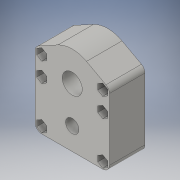
# Autodesk Inventor part: Transmission box
Saved by Autodesk Inventor 2016 SP2 (Build 200236200, 236)
## iProperties
Created: 2018-01-18
Part Number: Transmission box
Material: Generic
Document SubType Name: Modeling
Designer: CAD
Density: 1 g/cm^3
Appearance: Default
Author: CAD
Autodesk Inventor part; units mm, degrees
ref_plane "YZ Plane" through (0, 0, 0) normal (1, 0, 0) x (0, 1, 0)
ref_plane "XZ Plane" through (0, 0, 0) normal (0, 1, 0) x (-1, 0, 0)
ref_plane "XY Plane" through (0, 0, 0) normal (0, 0, 1) x (1, 0, 0)
sketch "Sketch1" plane through (0, 0, 0) normal (0, 0, 1) x (1, 0, 0)
  line L0 (9.525, 0) -> (96.8375, 0)
  arc A0 (0, 9.525) -> (9.525, 0) centre (9.525, 9.525) ccw
  arc A1 (96.8375, 0) -> (106.3625, 9.525) centre (96.8375, 9.525) ccw
  arc A2 (106.3625, 98.425) -> (101.3693, 106.8029) centre (96.8375, 98.425) ccw
  circle A3 centre (53.1813, 84.1375) radius 14.2875
  line L1 (32.7882, 121.8379) -> (4.9932, 106.8029)
  line L2 (73.5743, 121.8379) -> (101.3693, 106.8029)
  line L3 (0, 98.425) -> (0, 9.525)
  line L4 (106.3625, 9.525) -> (106.3625, 98.425)
  arc A4 (73.5743, 121.8379) -> (32.7882, 121.8379) centre (53.1813, 84.1375) ccw
  arc A5 (4.9932, 106.8029) -> (0, 98.425) centre (9.525, 98.425) ccw
  point P0 (0, 0)
  constraints: 10 end point, 10 point on circle, 6 centre point, 5 tangent, 1 coincident, 1 horizontal
extrude "Extrusion1" add sketch "Sketch1" along normal blind 50.8
sketch "Sketch2" plane through (0, 0, 50.8) normal (0, 0, 1) x (1, 0, 0)
  arc A0 (0, 9.525) -> (9.525, 0) centre (9.525, 9.525) ccw projected
  arc A1 (96.8375, 0) -> (106.3625, 9.525) centre (96.8375, 9.525) ccw projected
  line L0 (96.8375, 0) -> (96.8375, 9.525)
  arc A2 (106.3625, 98.425) -> (101.3693, 106.8029) centre (96.8375, 98.425) ccw projected
  line L1 (106.3625, 98.425) -> (96.8375, 98.425)
  arc A3 (4.9932, 106.8029) -> (0, 98.425) centre (9.525, 98.425) ccw projected
  line L2 (9.525, 90.1761) -> (9.525, 79.0636)
  line L3 (2.3813, 94.7588) -> (2.3812, 102.0912)
  line L4 (9.525, 84.6199) -> (12.0788, 84.6199)
  line L5 (0, 9.525) -> (0, 53.975)
  line L6 (0, 53.975) -> (101.6, 53.975)
  circle A4 centre (53.1813, 84.1375) radius 14.2875 projected
  line L7 (53.1813, 84.1375) -> (53.1813, -32.9596)
  line L8 (9.525, 98.425) -> (2.3813, 98.425)
  line L9 (2.3813, 102.5494) -> (9.525, 106.6739)
  line L10 (9.525, 106.6739) -> (16.6687, 102.5494)
  line L11 (16.6687, 102.5494) -> (16.6687, 94.3006)
  line L12 (16.6687, 94.3006) -> (9.525, 90.1761)
  line L13 (9.525, 90.1761) -> (2.3813, 94.3006)
  line L14 (2.3813, 94.3006) -> (2.3813, 102.5494)
  line L15 (2.3813, 74.4809) -> (2.3812, 67.1485)
  line L16 (9.525, 70.8147) -> (2.3813, 70.8147)
  line L17 (2.3813, 66.6903) -> (9.525, 62.5658)
  line L18 (9.525, 62.5658) -> (16.6687, 66.6903)
  line L19 (16.6687, 66.6903) -> (16.6687, 74.9392)
  line L20 (16.6687, 74.9392) -> (9.525, 79.0636)
  line L21 (9.525, 79.0636) -> (2.3813, 74.9392)
  line L22 (2.3813, 74.9392) -> (2.3813, 66.6903)
  arc A5 (0, 9.525) -> (4.9932, 1.1471) centre (9.525, 9.525) ccw
  line L23 (2.3813, 13.1912) -> (2.3812, 5.8588)
  line L24 (9.525, 9.525) -> (2.3813, 9.525)
  line L25 (2.3813, 5.4006) -> (9.525, 1.2761)
  line L26 (9.525, 1.2761) -> (16.6687, 5.4006)
  line L27 (16.6687, 5.4006) -> (16.6687, 13.6494)
  line L28 (16.6687, 13.6494) -> (9.525, 17.7739)
  line L29 (9.525, 17.7739) -> (2.3813, 13.6494)
  line L30 (2.3813, 13.6494) -> (2.3813, 5.4006)
  line L31 (96.8375, 90.1761) -> (96.8375, 79.0636)
  line L32 (103.9813, 94.7588) -> (103.9813, 102.0912)
  line L33 (96.8375, 84.6199) -> (94.2837, 84.6199)
  line L34 (96.8375, 98.425) -> (103.9813, 98.425)
  line L35 (103.9813, 102.5494) -> (96.8375, 106.6739)
  line L36 (96.8375, 106.6739) -> (89.6938, 102.5494)
  line L37 (89.6938, 102.5494) -> (89.6938, 94.3006)
  line L38 (89.6938, 94.3006) -> (96.8375, 90.1761)
  line L39 (96.8375, 90.1761) -> (103.9813, 94.3006)
  line L40 (103.9813, 94.3006) -> (103.9813, 102.5494)
  line L41 (89.6938, 66.6903) -> (89.6938, 74.9392)
  line L42 (96.8375, 62.5658) -> (89.6938, 66.6903)
  line L43 (89.6938, 74.9392) -> (96.8375, 79.0636)
  line L44 (96.8375, 70.8147) -> (103.9813, 70.8147)
  line L45 (103.9813, 74.4809) -> (103.9813, 67.1485)
  line L46 (96.8375, 79.0636) -> (103.9813, 74.9392)
  line L47 (103.9813, 74.9392) -> (103.9813, 66.6903)
  line L48 (103.9813, 66.6903) -> (96.8375, 62.5658)
  line L49 (96.8375, 1.2761) -> (89.6938, 5.4006)
  line L50 (89.6938, 5.4006) -> (89.6938, 13.6494)
  line L51 (89.6938, 13.6494) -> (96.8375, 17.7739)
  line L52 (96.8375, 17.7739) -> (103.9813, 13.6494)
  line L53 (96.8375, 9.525) -> (103.9813, 9.525)
  line L54 (103.9813, 5.4006) -> (96.8375, 1.2761)
  line L55 (103.9813, 13.1912) -> (103.9813, 5.8588)
  arc A6 (101.3693, 1.1471) -> (106.3625, 9.525) centre (96.8375, 9.525) ccw
  line L56 (103.9813, 13.6494) -> (103.9813, 5.4006)
  point P0 (0, 0)
  point P1 (96.8375, 9.525)
  point P2 (96.8375, 98.425)
  point P3 (96.8375, 9.525)
  dimension "d15" = 11.1125
  constraints: 114 end point, 60 symmetric about line, 6 coincident, 4 point on circle, 3 horizontal, 3 midpoint, 3 vertical, 2 centre point, 15 other
  measures "d15" distance of L2.start L2.end
extrude "Extrusion2" cut sketch "Sketch2" against normal through all contours L49 L50 L51 L52 L56 L55 L53 L0 | L0 L53 L55 L56 L54 | L20 L19 L18 L17 L22 L15 L21 | L13 L14 L3 L9 L10 L11 L12 | L30 L29 L28 L27 L26 L25 L23 | L46 L47 L45 L48 L42 L41 L43 | L38 L37 L36 L35 L40 L32 L39
sketch "Sketch3" plane through (0, 0, 50.8) normal (0, 0, 1) x (1, 0, 0)
  circle A0 centre (53.1813, 31.75) radius 9.525
  circle A1 centre (53.1813, 84.1375) radius 14.2875 projected
  line L0 (53.1813, 69.85) -> (53.1813, 31.75)
  point P0 (0, 0)
  dimension "d25" = 19.05
  dimension "d27" = 38.1
  constraints: 2 end point, 1 centre point, 1 vertical, 1 vertical alignment, 1 other
  measures "d25" diameter of A0
  measures "d27" distance of L0.start L0.end
extrude "Extrusion3" cut sketch "Sketch3" against normal through all contours A0
body "Solid1"
